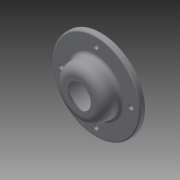
# Autodesk Inventor part: supportoCuscinettoBasso
Saved by Autodesk Inventor 2014 SP2 (Build 180246200, 246)
## iProperties
Created: 2019-05-08
Part Number: supportoCuscinettoBasso
Material: Generic
Document SubType Name: Modeling
Designer: GauchoHP
Density: 1 g/cm^3
Appearance: Default
Author: GauchoHP
Autodesk Inventor part; units mm, degrees
ref_plane "YZ Plane" through (0, 0, 0) normal (1, 0, 0) x (0, 1, 0)
ref_plane "XZ Plane" through (0, 0, 0) normal (0, 1, 0) x (-1, 0, 0)
ref_plane "XY Plane" through (0, 0, 0) normal (0, 0, 1) x (1, 0, 0)
sketch "Sketch1" plane through (0, 0, 0) normal (0, 1, 0) x (-1, 0, 0)
  circle A0 centre (0, 0) radius 11.25
  circle A1 centre (0, 0) radius 14.25
  circle A2 centre (0, 0) radius 30
  circle A3 centre (0, 0) radius 6.75
  dimension "d0" = 22.5
  dimension "d1" = 28.5
  dimension "d2" = 60
  dimension "d3" = 13.5
  constraints: 4 centre point, 4 coincident
  measures "d0" diameter of A0
  measures "d1" diameter of A1
  measures "d2" diameter of A2
  measures "d3" diameter of A3
extrude "Extrusion1" add sketch "Sketch1" along normal blind 4.5 contours A0 | A1
sketch "Sketch2" plane through (0, 4.5, 0) normal (0, 1, 0) x (1, 0, 0)
  circle A0 centre (0, 0) radius 14.25 projected
  circle A1 centre (0, 0) radius 11.25
  dimension "d6" = 22.5
  constraints: 1 centre point, 1 coincident
  measures "d6" diameter of A1
extrude "Extrusion2" add sketch "Sketch2" along normal blind 8
sketch "Sketch3" plane through (0, 12.5, 0) normal (0, 1, 0) x (1, 0, 0)
  circle A0 centre (0, 0) radius 14.25 projected
  circle A1 centre (0, 0) radius 25.25
  dimension "d9" = 50.5
  constraints: 1 centre point, 1 coincident
  measures "d9" diameter of A1
extrude "Extrusion3" add sketch "Sketch3" against normal blind 3
chamfer "Chamfer2" distance 4.5 angle 45 1 edges at (6.75, 4.5, 0)
fillet "Fillet1" radius 5 1 edges at (14.25, 0, 0)
fillet "Fillet2" radius 2 1 edges at (-14.25, 9.5, 0)
fillet "Fillet3" radius 1 1 edges at (-25.25, 9.5, 0)
sketch "Sketch5" plane through (0, 9.5, 0) normal (0, -1, 0) x (1, 0, 0)
  circle A0 centre (0, 0) radius 16.25 projected
  circle A1 centre (-20, 0) radius 1.5
  circle A2 centre (-20, 0) radius 3.75
  circle A3 centre (20, 0) radius 1.5
  circle A4 centre (0, -20) radius 1.5
  circle A5 centre (0, 20) radius 1.5
  dimension "d21" = 3
  dimension "d22" = 20
  dimension "d23" = 3
  dimension "d24" = 20
  dimension "d25" = 3
  dimension "d26" = 20
  dimension "d27" = 3
  dimension "d28" = 20
  constraints: 5 centre point, 1 coincident, 1 tangent
  measures "d21" diameter of A1
  measures "d22" distance of A0.centre A1.centre
  measures "d23" diameter of A3
  measures "d24" distance of A0.centre A3.centre
  measures "d25" diameter of A4
  measures "d26" distance of A0.centre A4.centre
  measures "d27" diameter of A5
  measures "d28" distance of A0.centre A5.centre
extrude "Extrusion4" cut sketch "Sketch5" against normal blind 11 contours A1 | A3 | A4 | A5
body "Solid1"
